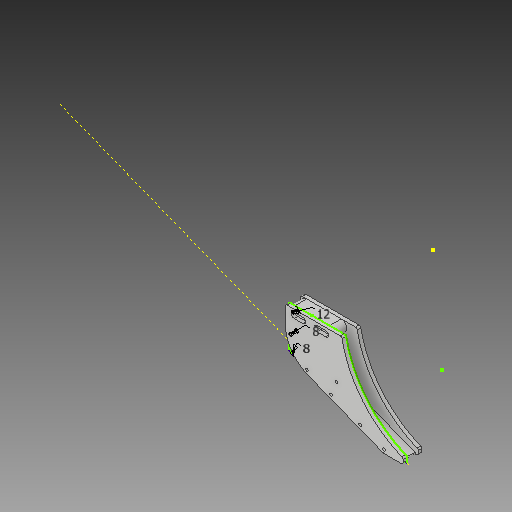
# Autodesk Inventor part: ChainGuide
Saved by Autodesk Inventor 2019.3 (Build 233278000, 278)
## iProperties
Created: 2019-02-13
Part Number: ChainGuide
Material: Generic
Document SubType Name: Modeling
Designer: eroldan
Density: 1 g/cm^3
Appearance: Default
Author: eroldan
Autodesk Inventor part; units mm, degrees
ref_plane "YZ Plane" through (0, 0, 0) normal (1, 0, 0) x (0, 1, 0)
ref_plane "XZ Plane" through (0, 0, 0) normal (0, 1, 0) x (-1, 0, 0)
ref_plane "XY Plane" through (0, 0, 0) normal (0, 0, 1) x (1, 0, 0)
sketch "Sketch1" plane through (0, 0, 0) normal (0, 0, 1) x (1, 0, 0)
  line L0 (-97.6616, -130.6576) -> (-160.8785, -130.6576)
  line L1 (-160.8785, -130.6576) -> (-160.8785, -176.6929)
  line L2 (-160.8785, -176.6929) -> (-50.8498, -220.1435)
  arc A0 (-97.6616, -130.6576) -> (-29.0692, -213.8163) centre (10.8943, -110.9847) ccw
  line L3 (-418.958, -66.1755) -> (-24.673, -221.8796) construction
  line L4 (-29.258, -220.0689) -> (-153.9234, -170.8383)
  line L5 (-156.8618, -178.2791) -> (-51.0386, -220.0689)
  arc A1 (-153.9234, -170.8383) -> (-156.8618, -178.2791) centre (-155.3926, -174.5587) ccw
  line L6 (-29.258, -220.0689) -> (-51.0386, -220.0689)
  line L7 (-50.8498, -220.1435) -> (-29.0692, -220.1435)
  line L8 (-29.0692, -213.8163) -> (-29.0692, -220.1435)
  line L9 (-115.2361, -136.6576) -> (-153.9234, -136.6576) construction
  line L10 (-115.2361, -130.6576) -> (-153.9234, -130.6576)
  line L11 (-153.9234, -142.6576) -> (-115.2361, -142.6576)
  arc A2 (-115.2361, -142.6576) -> (-115.2361, -130.6576) centre (-115.2361, -136.6576) ccw
  arc A3 (-153.9234, -130.6576) -> (-153.9234, -142.6576) centre (-153.9234, -136.6576) ccw
  line L12 (-103.5313, -177.5782) -> (-155.3714, -157.446) construction
  line L13 (-102.0833, -173.8495) -> (-153.9234, -153.7173)
  line L14 (-156.8195, -161.1747) -> (-104.9794, -181.3069)
  arc A4 (-104.9794, -181.3069) -> (-102.0833, -173.8495) centre (-103.5313, -177.5782) ccw
  arc A5 (-153.9234, -153.7173) -> (-156.8195, -161.1747) centre (-155.3714, -157.446) ccw
  point P0 (0, 0)
  point P1 (-134.5797, -136.6576)
  point P2 (-129.4514, -167.5121)
  point P3 (-134.5797, -130.6576)
  dimension "d6" = 12
  dimension "d8" = 8
  dimension "d9" = 8
  constraints: 32 end point, 12 point on circle, 10 tangent, 6 centre point, 4 parallel, 3 collinear, 3 horizontal, 3 midpoint, 2 point on line, 1 perpendicular, 1 vertical
  measures "d6" diameter of A3
  measures "d8" diameter of A1
  measures "d9" diameter of A5
extrude "Extrusion2" add sketch "Sketch1" along normal blind 4 contours A0 L8 L7 L2 L6 L4 A1 L1 L0 A3 L11 A2 | A2 L11 A3 L0 | L2 A1 L4 L6 | A4 L14 A5 L13
fillet "Fillet4" radius 40 1 edges at (-160.8785, -176.6929, 2)
sketch "Sketch8" plane through (0, 0, 0) normal (0, 0, -1) x (-1, 0, 0)
  arc A0 (135.5705, -186.6871) -> (160.8785, -149.483) centre (120.8785, -149.483) ccw projected
  line L0 (160.8785, -149.483) -> (160.8785, -130.6576) projected
  line L1 (160.8785, -130.6576) -> (97.6616, -130.6576) projected
  arc A1 (29.0692, -213.8163) -> (97.6616, -130.6576) centre (-10.8943, -110.9847) ccw projected
  line L2 (29.0692, -213.8163) -> (29.0692, -220.1435) projected
  line L3 (29.0692, -220.1435) -> (50.8498, -220.1435) projected
  line L4 (50.8498, -220.1435) -> (135.5705, -186.6871) projected
  line L5 (418.958, -66.1755) -> (24.673, -221.8796) projected
  line L6 (156.8618, -178.2791) -> (51.0386, -220.0689) projected
  line L7 (29.258, -220.0689) -> (51.0386, -220.0689) projected
  line L8 (156.8195, -161.1747) -> (104.9794, -181.3069) projected
  arc A2 (156.8195, -161.1747) -> (153.9234, -153.7173) centre (155.3714, -157.446) ccw projected
  line L9 (102.0833, -173.8495) -> (153.9234, -153.7173) projected
  arc A3 (102.0833, -173.8495) -> (104.9794, -181.3069) centre (103.5313, -177.5782) ccw projected
  line L10 (153.9234, -142.6576) -> (115.2361, -142.6576) projected
  arc A4 (115.2361, -130.6576) -> (115.2361, -142.6576) centre (115.2361, -136.6576) ccw projected
  line L11 (115.2361, -130.6576) -> (153.9234, -130.6576) projected
  arc A5 (153.9234, -142.6576) -> (153.9234, -130.6576) centre (153.9234, -136.6576) ccw projected
  arc A6 (135.5705, -186.6871) -> (160.8785, -149.483) centre (120.8785, -149.483) ccw projected
  arc A7 (135.5705, -186.6871) -> (154.9546, -170.431) centre (120.8785, -149.483) ccw
  point P0 (0, 0)
  constraints: 4 point on circle, 2 point on line, 1 centre point
extrude "Extrusion8" add sketch "Sketch8" along normal blind 13 separate body contours L4 L7 L5 A0 | A5 L10 A4 L1 | L8 A3 L9 A2
sketch "Sketch9" plane through (0, 0, -13) normal (0, 0, -1) x (-1, 0, 0)
  arc A0 (135.5705, -186.6871) -> (160.8785, -149.483) centre (120.8785, -149.483) ccw projected
  line L0 (135.5705, -186.6871) -> (50.8498, -220.1435) projected
  line L1 (50.8498, -220.1435) -> (29.0692, -220.1435) projected
  line L2 (29.0692, -220.1435) -> (29.0692, -213.8163) projected
  arc A1 (29.0692, -213.8163) -> (97.6616, -130.6576) centre (-10.8943, -110.9847) ccw projected
  line L3 (97.6616, -130.6576) -> (160.8785, -130.6576) projected
  line L4 (160.8785, -130.6576) -> (160.8785, -149.483) projected
  point P0 (0, 0)
extrude "Extrusion9" add sketch "Sketch9" along normal blind 4 separate body
fillet "Fillet5" radius 2 11 edges at (-160.8785, -130.6576, 2) (-97.6616, -130.6576, 2) (-29.0692, -213.8163, 2) (-29.0692, -220.1435, 2) (-50.8498, -220.1435, 2) (-51.0386, -220.0689, -6.5) (-160.8785, -130.6576, -15) (-97.6616, -130.6576, -15) (-29.0692, -213.8163, -15) (-29.0692, -220.1435, -15) (-50.8498, -220.1435, -15)
fillet "Fillet5" radius 0.75 1 edges at (-29.258, -220.0689, -6.5)
sketch "Sketch11" plane through (0, 0, -17) normal (0, 0, -1) x (-1, 0, 0)
  arc A0 (115.2361, -130.6576) -> (115.2361, -142.6576) centre (115.2361, -136.6576) ccw construction
  arc A1 (102.0833, -173.8495) -> (104.9794, -181.3069) centre (103.5313, -177.5782) ccw construction
  line L0 (154.9546, -170.431) -> (32.9237, -218.6213) construction
  line L1 (136.6088, -182.3122) -> (50.4178, -216.2223) construction
  line L2 (140.8742, -136.6576) -> (150.8742, -136.6576) construction
  line L3 (140.8742, -139.6576) -> (150.8742, -139.6576)
  line L4 (150.8742, -133.6576) -> (140.8742, -133.6576)
  arc A2 (140.8742, -133.6576) -> (140.8742, -139.6576) centre (140.8742, -136.6576) ccw
  arc A3 (150.8742, -139.6576) -> (150.8742, -133.6576) centre (150.8742, -136.6576) ccw
  line L5 (115.3787, -136.6576) -> (125.3787, -136.6576) construction
  line L6 (115.3787, -139.6576) -> (125.3787, -139.6576)
  line L7 (125.3787, -133.6576) -> (115.3787, -133.6576)
  arc A4 (115.3787, -133.6576) -> (115.3787, -139.6576) centre (115.3787, -136.6576) ccw
  arc A5 (125.3787, -139.6576) -> (125.3787, -133.6576) centre (125.3787, -136.6576) ccw
  arc A6 (156.8195, -161.1747) -> (153.9234, -153.7173) centre (155.3714, -157.446) ccw construction
  circle A7 centre (50.4178, -216.2223) radius 1.5
  circle A8 centre (77.1382, -205.7097) radius 1.5
  circle A9 centre (109.7086, -192.8956) radius 1.5
  circle A10 centre (136.6088, -182.3122) radius 1.5
  circle A11 centre (155.3714, -157.446) radius 1.5
  circle A12 centre (103.5313, -177.5782) radius 1.5
  point P0 (0, 0)
  point P1 (145.8742, -136.6576)
  point P2 (120.3787, -136.6576)
  dimension "d43" = 10
  dimension "d44" = 6
  dimension "d45" = 10
  dimension "d46" = 6
  dimension "d47" = 3
  dimension "d48" = 3
  dimension "d49" = 3
  dimension "d50" = 3
  dimension "d51" = 3
  dimension "d52" = 3
  constraints: 18 end point, 10 centre point, 8 coincident, 8 point on circle, 8 tangent, 2 midpoint, 2 parallel, 2 point on line, 1 horizontal
  measures "d43" distance of L2.start L2.end
  measures "d44" diameter of A3
  measures "d45" distance of L5.start L5.end
  measures "d46" diameter of A5
  measures "d47" diameter of A7
  measures "d48" diameter of A8
  measures "d49" diameter of A9
  measures "d50" diameter of A10
  measures "d51" diameter of A11
  measures "d52" diameter of A12
extrude "Extrusion10" cut sketch "Sketch11" against normal through all bodies 3 1 2
